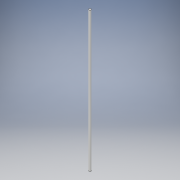
# Autodesk Inventor part: Rod Central
Saved by Autodesk Inventor 2019 (Build 230136000, 136)
## iProperties
Created: 2019-04-27
Part Number: Rod Central
Material: Generic
Document SubType Name: Modeling
Designer: isadmin
Density: 1 g/cm^3
Appearance: Default
Author: isadmin
Autodesk Inventor part; units mm, degrees
ref_plane "YZ Plane" through (0, 0, 0) normal (1, 0, 0) x (0, 1, 0)
ref_plane "XZ Plane" through (0, 0, 0) normal (0, 1, 0) x (-1, 0, 0)
ref_plane "XY Plane" through (0, 0, 0) normal (0, 0, 1) x (1, 0, 0)
sketch "Sketch1" plane through (0, 0, 0) normal (0, 0, 1) x (1, 0, 0)
  line L0 (-3.2147, 594.1219) -> (1.5478, 594.1219)
  line L1 (1.5478, 594.1219) -> (1.5478, -15.4781)
  line L2 (1.5478, -15.4781) -> (-3.2147, -15.4781)
  line L3 (-3.2147, -15.4781) -> (-3.2147, 594.1219)
  point P0 (0, 0)
  dimension "d1" = 4.7625
  dimension "d2" = 609.6
  constraints: 8 end point, 2 parallel, 1 horizontal, 1 perpendicular
  measures "d1" distance of L0.start L0.end
  measures "d2" distance of L0.end L1.end
revolve "Revolution1" add sketch "Sketch1" angle 360 about axis through (1.5478, 594.1219, 0) along (0, -1, 0)
body "Solid1"
